gear-wheel-41 v3 (Autodesk Fusion 360 design; units mm, degrees)
description: Spur Gear; Module: 0.3; Num Teeth: 41; Pressure Angle: 20.0; Backlash: 0.00 mm
Autodesk Fusion 360 part; units mm, degrees
sketch "スケッチ1" plane through (0, 0, 0) normal (0, 0, 1) x (1, 0, 0) in component "Spur Gear (41 teeth)"
  circle A0 centre (0, 0) radius 5.7392
  circle A1 centre (0, 0) radius 4.975
extrude "押し出し1" add sketch "スケッチ1" along normal blind 1 in component "Spur Gear (41 teeth)"
sketch "スケッチ2" plane through (0, 0, 0) normal (0, 0, 1) x (1, 0, 0) in component "Spur Gear (41 teeth)"
  spline S0 degree 5 poles (5.7709, -0.3074) (5.7729, -0.3075) (5.7767, -0.3076) (5.7826, -0.3077) (5.7903, -0.3076) (5.8, -0.3072) (5.8096, -0.3066) (5.8193, -0.3058) (5.829, -0.305) (5.8387, -0.304) (5.8484, -0.303) (5.8581, -0.3019) (5.8678, -0.3007) (5.8775, -0.2994) (5.8872, -0.298) (5.8969, -0.2965) (5.9067, -0.295) (5.9164, -0.2933) (5.9261, -0.2916) (5.9358, -0.2898) (5.9455, -0.2879) (5.9552, -0.286) (5.965, -0.284) (5.9747, -0.2819) (5.9844, -0.2797) (5.9941, -0.2775) (6.0038, -0.2753) (6.0136, -0.2729) (6.0233, -0.2705) (6.033, -0.2681) (6.0427, -0.2656) (6.0524, -0.263) (6.0621, -0.2604) (6.0719, -0.2577) (6.0816, -0.255) (6.0913, -0.2522) (6.101, -0.2493) (6.1107, -0.2464) (6.1204, -0.2434) (6.1301, -0.2404) (6.1398, -0.2374) (6.1495, -0.2343) (6.1592, -0.2311) (6.1689, -0.2279) (6.1786, -0.2246) (6.1883, -0.2213) (6.198, -0.218) (6.2077, -0.2145) (6.2174, -0.2111) (6.2271, -0.2076) (6.2368, -0.204) (6.2465, -0.2004) (6.2561, -0.1968) (6.2658, -0.1931) (6.2755, -0.1893) (6.2852, -0.1855) (6.2948, -0.1817) (6.3045, -0.1778) (6.3141, -0.1739) (6.3238, -0.1699) (6.3335, -0.1659) (6.3431, -0.1619) (6.3527, -0.1578) (6.3624, -0.1536) (6.372, -0.1494) (6.3817, -0.1452) (6.3913, -0.1409) (6.4009, -0.1366) (6.4105, -0.1322) (6.4202, -0.1278) (6.4298, -0.1234) (6.4375, -0.1198) (6.4432, -0.1171) (6.4471, -0.1153) (6.449, -0.1144) knots 0 0 0 0 0 0 0.01428571 0.02857143 0.04285714 0.05714286 0.07142857 0.08571429 0.1 0.11428571 0.12857143 0.14285714 0.15714286 0.17142857 0.18571429 0.2 0.21428571 0.22857143 0.24285714 0.25714286 0.27142857 0.28571429 0.3 0.31428571 0.32857143 0.34285714 0.35714286 0.37142857 0.38571429 0.4 0.41428571 0.42857143 0.44285714 0.45714286 0.47142857 0.48571429 0.5 0.51428571 0.52857143 0.54285714 0.55714286 0.57142857 0.58571429 0.6 0.61428571 0.62857143 0.64285714 0.65714286 0.67142857 0.68571429 0.7 0.71428571 0.72857143 0.74285714 0.75714286 0.77142857 0.78571429 0.8 0.81428571 0.82857143 0.84285714 0.85714286 0.87142857 0.88571429 0.9 0.91428571 0.92857143 0.94285714 0.95714286 0.97142857 0.98571429 1 1 1 1 1 1
  spline S1 degree 5 poles (5.7709, 0.3074) (5.7729, 0.3075) (5.7767, 0.3076) (5.7826, 0.3077) (5.7903, 0.3076) (5.8, 0.3072) (5.8096, 0.3066) (5.8193, 0.3058) (5.829, 0.305) (5.8387, 0.304) (5.8484, 0.303) (5.8581, 0.3019) (5.8678, 0.3007) (5.8775, 0.2994) (5.8872, 0.298) (5.8969, 0.2965) (5.9067, 0.295) (5.9164, 0.2933) (5.9261, 0.2916) (5.9358, 0.2898) (5.9455, 0.2879) (5.9552, 0.286) (5.965, 0.284) (5.9747, 0.2819) (5.9844, 0.2797) (5.9941, 0.2775) (6.0038, 0.2753) (6.0136, 0.2729) (6.0233, 0.2705) (6.033, 0.2681) (6.0427, 0.2656) (6.0524, 0.263) (6.0621, 0.2604) (6.0719, 0.2577) (6.0816, 0.255) (6.0913, 0.2522) (6.101, 0.2493) (6.1107, 0.2464) (6.1204, 0.2434) (6.1301, 0.2404) (6.1398, 0.2374) (6.1495, 0.2343) (6.1592, 0.2311) (6.1689, 0.2279) (6.1786, 0.2246) (6.1883, 0.2213) (6.198, 0.218) (6.2077, 0.2145) (6.2174, 0.2111) (6.2271, 0.2076) (6.2368, 0.204) (6.2465, 0.2004) (6.2561, 0.1968) (6.2658, 0.1931) (6.2755, 0.1893) (6.2852, 0.1855) (6.2948, 0.1817) (6.3045, 0.1778) (6.3141, 0.1739) (6.3238, 0.1699) (6.3335, 0.1659) (6.3431, 0.1619) (6.3527, 0.1578) (6.3624, 0.1536) (6.372, 0.1494) (6.3817, 0.1452) (6.3913, 0.1409) (6.4009, 0.1366) (6.4105, 0.1322) (6.4202, 0.1278) (6.4298, 0.1234) (6.4375, 0.1198) (6.4432, 0.1171) (6.4471, 0.1153) (6.449, 0.1144) knots 0 0 0 0 0 0 0.01428571 0.02857143 0.04285714 0.05714286 0.07142857 0.08571429 0.1 0.11428571 0.12857143 0.14285714 0.15714286 0.17142857 0.18571429 0.2 0.21428571 0.22857143 0.24285714 0.25714286 0.27142857 0.28571429 0.3 0.31428571 0.32857143 0.34285714 0.35714286 0.37142857 0.38571429 0.4 0.41428571 0.42857143 0.44285714 0.45714286 0.47142857 0.48571429 0.5 0.51428571 0.52857143 0.54285714 0.55714286 0.57142857 0.58571429 0.6 0.61428571 0.62857143 0.64285714 0.65714286 0.67142857 0.68571429 0.7 0.71428571 0.72857143 0.74285714 0.75714286 0.77142857 0.78571429 0.8 0.81428571 0.82857143 0.84285714 0.85714286 0.87142857 0.88571429 0.9 0.91428571 0.92857143 0.94285714 0.95714286 0.97142857 0.98571429 1 1 1 1 1 1
  arc A0 (6.449, -0.1144) -> (6.449, 0.1144) centre (0, 0) ccw
  line L0 (5.7211, -0.3053) -> (5.7709, -0.3074)
  line L1 (5.7211, 0.3053) -> (5.7709, 0.3074)
  line L2 (5.7211, -0.3053) -> (5.7211, 0.3053)
  point P0 (5.819, -0.3058)
  point P1 (5.8672, -0.3008)
  point P2 (5.9156, -0.2934)
  point P3 (5.964, -0.2841)
  point P4 (6.0125, -0.2732)
  point P5 (6.061, -0.2607)
  point P6 (6.1096, -0.2467)
  point P7 (6.1581, -0.2315)
  point P8 (6.2067, -0.2149)
  point P9 (6.2552, -0.1971)
  point P10 (6.3037, -0.1781)
  point P11 (6.3522, -0.158)
  point P12 (6.4006, -0.1367)
  point P13 (5.819, 0.3058)
  point P14 (5.8672, 0.3008)
  point P15 (5.9156, 0.2934)
  point P16 (5.964, 0.2841)
  point P17 (6.0125, 0.2732)
  point P18 (6.061, 0.2607)
  point P19 (6.1096, 0.2467)
  point P20 (6.1581, 0.2315)
  point P21 (6.2067, 0.2149)
  point P22 (6.2552, 0.1971)
  point P23 (6.3037, 0.1781)
  point P24 (6.3522, 0.158)
  point P25 (6.4006, 0.1367)
extrude "押し出し2" add sketch "スケッチ2" along normal blind 1 in component "Spur Gear (41 teeth)"
pattern_circular "C パターン1" count 41 over 360 about axis through (0, 0, 0) along (0, 0, 1) of "押し出し2" in component "Spur Gear (41 teeth)"
sketch "スケッチ3" plane through (0, 0, 0) normal (0, 0, 1) x (1, 0, 0) in component "Spur Gear (41 teeth)"
  circle A0 centre (0, 0) radius 6.15 construction
component "Spur Gear (41 teeth)" placed x (1, 0, 0) y (0, 1, 0) z (0, 0, 1) at (0, 0, 0)
